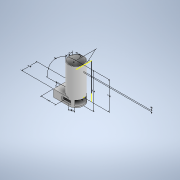
# Autodesk Inventor part: HousingMKII
Saved by Autodesk Inventor 2021 (Build 250183000, 183)
## iProperties
Created: 2020-06-26
Part Number: HousingMKII
Material: Generic
Document SubType Name: Modeling
Designer: Jaysonn
Density: 1 g/cm^3
Appearance: Default
Author: Jaysonn
## iProperties of the stored document _3DPrint.ipt
Created: 2020-06-26
Part Number: _3DPrint
Material: Generic
Document SubType Name: Modeling
Designer: Jaysonn
Density: 1 g/cm^3
Appearance: Default
Author: Jaysonn
Autodesk Inventor part; units mm, degrees
ref_plane "XZ Plane" through (0, 0, 0) normal (0, 1, 0) x (-1, 0, 0)
ref_plane "XY Plane" through (0, 0, 0) normal (0, 0, 1) x (1, 0, 0)
sketch "Sketch1" plane through (0, 0, 0) normal (0, 0, 1) x (1, 0, 0)
  point P0 (0, 0)
sketch "Sketch2" plane through (0, 0, 0) normal (0, 1, 0) x (-1, 0, 0)
  circle A0 centre (0, 0) radius 34.29
  dimension "d0" = 68.58
  constraints: 1 centre point, 1 coincident
  measures "d0" diameter of A0
extrude "BaseCup" add sketch "Sketch2" along normal blind 127
sketch "Sketch3" plane through (0, 127, 0) normal (0, 1, 0) x (1, 0, 0)
  circle A0 centre (0, 0) radius 31.75
  dimension "d3" = 63.5
  constraints: 1 centre point, 1 coincident
  measures "d3" diameter of A0
extrude "Extrusion2" cut sketch "Sketch3" against normal blind 134.9375
sketch "Sketch4" plane through (0, 0, 0) normal (0, -1, 0) x (1, 0, 0)
  circle A0 centre (0, 0) radius 34.29
  dimension "d6" = 68.58
  constraints: 1 centre point, 1 coincident
  measures "d6" diameter of A0
extrude "Extrusion3" add sketch "Sketch4" along normal blind 33.02
ref_plane "Work Plane1" through (34.29, 0, 0) normal (1, 0, 0) x (0, 1, 0)
sketch "Sketch5" plane through (34.29, 0, 0) normal (1, 0, 0) x (0, 1, 0)
  point P0 (0, 0)
sketch "Sketch6" plane through (34.29, 0, 0) normal (1, 0, 0) x (0, 1, 0)
  line L0 (-3.5517, 27.0467) -> (-27.6817, 27.0467)
  line L1 (-27.6817, 27.0467) -> (-27.6817, -30.1033)
  line L2 (-27.6817, -30.1033) -> (-3.5517, -30.1033)
  line L3 (-3.5517, -30.1033) -> (-3.5517, 27.0467)
  point P0 (0, 0)
  dimension "d10" = 24.13
  dimension "d11" = 57.15
  constraints: 8 end point, 2 parallel, 1 horizontal, 1 perpendicular
  measures "d10" distance of L2.end L1.end
  measures "d11" distance of L1.end L0.end
extrude "Extrusion4" cut sketch "Sketch6" against normal blind 229.87
sketch "Sketch9" plane through (0, 0, 0) normal (1, 0, 0) x (0, 1, 0)
  line L0 (-33.02, 34.29) -> (127, 34.29) projected
  line L1 (-33.02, 34.29) -> (-33.02, -34.29) projected
  line L2 (0, 34.29) -> (-33.02, 34.29)
  line L3 (-33.02, 34.29) -> (-33.02, -34.29)
  line L4 (-33.02, -34.29) -> (0, -34.29)
  line L5 (0, -34.29) -> (0, 34.29)
  point P0 (0, 0)
  constraints: 8 end point, 2 parallel, 1 horizontal, 1 perpendicular, 1 point on line
extrude "Extrusion5" add sketch "Sketch9" against normal blind 67.31
sketch "Sketch10" plane through (34.29, 0, 0) normal (1, 0, 0) x (0, 1, 0)
  line L0 (-3.5517, 27.0467) -> (-3.5517, -30.1033) projected
  line L1 (-3.5517, 27.0467) -> (-27.6817, 27.0467)
  line L2 (-27.6817, 27.0467) -> (-27.6817, -30.1033)
  line L3 (-27.6817, -30.1033) -> (-3.5517, -30.1033)
  line L4 (-3.5517, -30.1033) -> (-3.5517, 27.0467)
  point P0 (0, 0)
  constraints: 8 end point, 2 parallel, 1 horizontal, 1 perpendicular
extrude "Extrusion6" cut sketch "Sketch10" against normal blind 99.3775
sketch "Sketch11" plane through (0, 0, 0) normal (0, 0, 1) x (1, 0, 0)
  line L0 (34.29, -3.5517) -> (16.4193, -3.5517) projected
  line L1 (34.29, -3.5517) -> (8.89, -3.5517)
  line L2 (8.89, -8.5174) -> (-29.21, -8.5174)
  line L3 (-29.21, -8.5174) -> (-29.21, -23.7574)
  line L4 (-29.21, -23.7574) -> (8.89, -23.7574)
  line L5 (8.89, -23.7574) -> (8.89, -8.5174)
  point P0 (0, 0)
  point P1 (21.078, -3.5517)
  dimension "d19" = 25.4
  dimension "d20" = 38.1
  dimension "d21" = 15.24
  constraints: 10 end point, 2 parallel, 1 collinear, 1 horizontal, 1 perpendicular
  measures "d19" distance of L0.start L1.end
  measures "d20" distance of L4.end L3.end
  measures "d21" distance of L3.end L2.end
extrude "Extrusion7" cut sketch "Sketch11" along normal blind 86.36
sketch "Sketch12" plane through (34.29, 0, 0) normal (1, 0, 0) x (0, 1, 0)
  line L0 (127, -34.29) -> (127, 34.29) projected
  line L1 (-33.02, -34.29) -> (0, -34.29) projected
  line L2 (127, -34.29) -> (0, -34.29)
  point P0 (0, 0)
  constraints: 2 end point, 1 collinear
sketch "Sketch13" plane through (0, 0, 0) normal (0, 1, 0) x (-1, 0, 0)
  point P0 (0, 0)
sketch "Sketch14" plane through (0, 0, 0) normal (1, 0, 0) x (0, 1, 0)
  line L0 (127.079, 0) -> (101.679, 0)
  line L1 (101.679, 0) -> (101.679, 15.24)
  line L2 (101.679, 15.24) -> (96.599, 15.24)
  line L3 (96.599, 15.24) -> (96.599, 17.78)
  line L4 (96.599, 17.78) -> (101.679, 17.78)
  line L5 (101.679, 17.78) -> (101.679, 15.24)
  line L6 (47.4963, 15.24) -> (42.4163, 15.24)
  line L7 (42.4163, 15.24) -> (42.4163, 17.78)
  line L8 (42.4163, 17.78) -> (47.4963, 17.78)
  line L9 (47.4963, 17.78) -> (47.4963, 15.24)
  line L10 (101.679, 0) -> (101.679, -15.24)
  line L11 (101.679, -15.24) -> (96.599, -15.24)
  line L12 (96.599, -15.24) -> (96.599, -17.78)
  line L13 (96.599, -17.78) -> (101.679, -17.78)
  line L14 (101.679, -17.78) -> (101.679, -15.24)
  line L15 (47.4963, -17.78) -> (42.4163, -17.78)
  line L16 (42.4163, -17.78) -> (42.4163, -15.24)
  line L17 (42.4163, -15.24) -> (47.4963, -15.24)
  line L18 (47.4963, -15.24) -> (47.4963, -17.78)
  point P0 (0, 0)
  dimension "d26" = 25.4
  dimension "d27" = 15.24
  dimension "d28" = 5.08
  dimension "d29" = 2.54
  dimension "d30" = 5.08
  dimension "d31" = 2.54
  dimension "d32" = 15.24
  dimension "d33" = 5.08
  dimension "d34" = 2.54
  constraints: 38 end point, 8 parallel, 5 horizontal, 5 perpendicular, 3 point on line, 1 vertical
  measures "d26" distance of L0.start L0.end
  measures "d27" distance of L0.end L1.end
  measures "d28" distance of L3.end L4.end
  measures "d29" distance of L2.end L3.end
  measures "d30" distance of L7.end L8.end
  measures "d31" distance of L6.end L7.end
  measures "d32" distance of L0.end L10.end
  measures "d33" distance of L13.end L12.end
  measures "d34" distance of L12.end L11.end
extrude "Extrusion8" cut sketch "Sketch14" against normal blind 99.06
sketch "Sketch15" plane through (0, 0, 0) normal (0, 0, 1) x (1, 0, 0)
  line L0 (0, 25.4328) -> (-17.78, 25.4328)
  line L1 (-17.78, 25.4328) -> (-17.78, 2.5728)
  line L2 (-17.78, 2.5728) -> (0, 2.5728)
  line L3 (0, 2.5728) -> (0, 25.4328)
  point P0 (0, 0)
  dimension "d37" = 17.78
  dimension "d38" = 22.86
  constraints: 8 end point, 2 parallel, 1 horizontal, 1 perpendicular
  measures "d37" distance of L2.end L1.end
  measures "d38" distance of L1.end L0.end
extrude "Extrusion9" cut sketch "Sketch15" against normal blind 99.06
body "Solid1"
